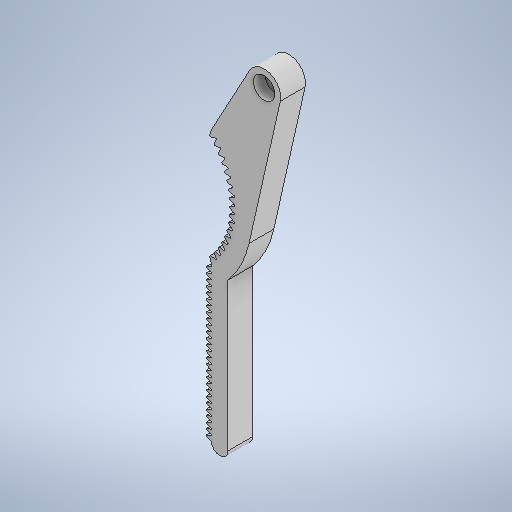
# Autodesk Inventor part: gripper_V2
Saved by Autodesk Inventor 2026.1 (Build 301233000, 233)
## iProperties
Created: 2025-11-11
Part Number: gripper_V2
Material: Generic
Document SubType Name: Modeling
Designer: kryst
Density: 1 g/cm^3
Appearance: Default
Author: kryst
Autodesk Inventor part; units mm, degrees
ref_plane "YZ Plane" through (0, 0, 0) normal (1, 0, 0) x (0, 1, 0)
ref_plane "XZ Plane" through (0, 0, 0) normal (0, 1, 0) x (-1, 0, 0)
ref_plane "XY Plane" through (0, 0, 0) normal (0, 0, 1) x (1, 0, 0)
sketch "Sketch1" plane through (0, 0, 0) normal (0, 0, 1) x (1, 0, 0)
  circle A0 centre (0, 0) radius 1.7
  circle A1 centre (0, 0) radius 3.25
  arc A2 (4.8776, -1.0993) -> (-4.3946, 2.3849) centre (0, 0) ccw
  line L0 (-16, -19) -> (-4.3946, 2.3849)
  arc A3 (-16, -54) -> (-16, -19) centre (-33.8536, -36.5) ccw
  line L1 (4.8776, -1.0993) -> (-4.5877, -43.096)
  line L2 (-10.3536, -36.25) -> (-10.3536, -36.75)
  line L3 (-10.3536, -36.75) -> (-8.8736, -37.5)
  line L4 (-10.3536, -36.25) -> (-8.8736, -35.5)
  line L5 (-10.475, -34.1008) -> (-9.0699, -33.2185)
  line L6 (-10.475, -34.1008) -> (-10.4293, -34.5987)
  line L7 (-10.4293, -34.5987) -> (-8.8869, -35.2101)
  line L8 (-10.4293, -38.4013) -> (-8.8869, -37.7899)
  line L9 (-10.4293, -38.4013) -> (-10.475, -38.8992)
  line L10 (-10.475, -38.8992) -> (-9.0699, -39.7815)
  line L11 (-10.7926, -31.9717) -> (-9.4741, -30.9645)
  line L12 (-10.7926, -31.9717) -> (-10.7015, -32.4633)
  line L13 (-10.7015, -32.4633) -> (-9.1096, -32.931)
  line L14 (-10.7015, -40.5367) -> (-9.1096, -40.069)
  line L15 (-10.7015, -40.5367) -> (-10.7926, -41.0283)
  line L16 (-10.7926, -41.0283) -> (-9.4741, -42.0355)
  line L17 (-11.3037, -29.8805) -> (-10.0829, -28.757)
  line L18 (-11.3037, -29.8805) -> (-11.168, -30.3618)
  line L19 (-11.168, -30.3618) -> (-9.54, -30.6819)
  line L20 (-11.168, -42.6382) -> (-9.54, -42.3181)
  line L21 (-11.168, -42.6382) -> (-11.3037, -43.1195)
  line L22 (-11.3037, -43.1195) -> (-10.0829, -44.243)
  line L23 (-12.004, -27.845) -> (-10.8911, -26.6144)
  line L24 (-12.004, -27.845) -> (-11.8248, -28.3117)
  line L25 (-11.8248, -28.3117) -> (-10.1744, -28.4816)
  line L26 (-11.8248, -44.6883) -> (-10.1744, -44.5184)
  line L27 (-11.8248, -44.6883) -> (-12.004, -45.155)
  line L28 (-12.004, -45.155) -> (-10.8911, -46.3856)
  line L29 (-12.8876, -25.882) -> (-11.892, -24.5548)
  line L30 (-12.8876, -25.882) -> (-12.6665, -26.3304)
  line L31 (-12.6665, -26.3304) -> (-11.0074, -26.3485)
  line L32 (-12.6665, -46.6696) -> (-11.0074, -46.6515)
  line L33 (-12.6665, -46.6696) -> (-12.8876, -47.118)
  line L34 (-12.8876, -47.118) -> (-11.892, -48.4452)
  line L35 (-13.9472, -24.0081) -> (-13.0771, -22.5954)
  line L36 (-13.9472, -24.0081) -> (-13.6859, -24.4344)
  line L37 (-13.6859, -24.4344) -> (-12.0321, -24.3006)
  line L38 (-13.6859, -48.5656) -> (-12.0321, -48.6994)
  line L39 (-13.6859, -48.5656) -> (-13.9472, -48.9919)
  line L40 (-13.9472, -48.9919) -> (-13.0771, -50.4047)
  line L41 (-15.1737, -22.2391) -> (-14.4366, -20.7526)
  line L42 (-15.1737, -22.2391) -> (-14.8745, -22.6397)
  line L43 (-14.8745, -22.6397) -> (-13.2399, -22.3551)
  line L44 (-14.8745, -50.3603) -> (-13.2399, -50.6449)
  line L45 (-14.8745, -50.3603) -> (-15.1737, -50.7609)
  line L46 (-15.1737, -50.7609) -> (-14.4366, -52.2474)
  line L47 (-16.557, -20.5896) -> (-15.9589, -19.042)
  line L48 (-16.557, -20.5896) -> (-16.2224, -20.9612)
  line L49 (-16.2224, -20.9612) -> (-14.6207, -20.5283)
  line L50 (-16.2224, -52.0388) -> (-14.6207, -52.4717)
  line L51 (-16.2224, -52.0388) -> (-16.557, -52.4104)
  line L52 (-16.557, -52.4104) -> (-15.9589, -53.958)
  line L53 (-15.9589, -53.958) -> (-15.9589, -100.657)
  line L54 (-15.9589, -53.958) -> (30.74, -53.958) construction
  arc A4 (-15.9589, -100.657) -> (-10.9589, -100.657) centre (-13.4589, -100.657) ccw
  line L55 (-17.4589, -99.732) -> (-17.4589, -100.082)
  line L56 (-17.4589, -100.082) -> (-15.9589, -100.657)
  line L57 (-17.4589, -99.732) -> (-15.9589, -99.157)
  line L58 (-17.4589, -98.032) -> (-15.9589, -97.457)
  line L59 (-17.4589, -98.032) -> (-17.4589, -98.382)
  line L60 (-17.4589, -98.382) -> (-15.9589, -98.957)
  line L61 (-17.4589, -96.332) -> (-15.9589, -95.757)
  line L62 (-17.4589, -96.332) -> (-17.4589, -96.682)
  line L63 (-17.4589, -96.682) -> (-15.9589, -97.257)
  line L64 (-17.4589, -94.632) -> (-15.9589, -94.057)
  line L65 (-17.4589, -94.632) -> (-17.4589, -94.982)
  line L66 (-17.4589, -94.982) -> (-15.9589, -95.557)
  line L67 (-17.4589, -92.932) -> (-15.9589, -92.357)
  line L68 (-17.4589, -92.932) -> (-17.4589, -93.282)
  line L69 (-17.4589, -93.282) -> (-15.9589, -93.857)
  line L70 (-17.4589, -91.232) -> (-15.9589, -90.657)
  line L71 (-17.4589, -91.232) -> (-17.4589, -91.582)
  line L72 (-17.4589, -91.582) -> (-15.9589, -92.157)
  line L73 (-17.4589, -89.532) -> (-15.9589, -88.957)
  line L74 (-17.4589, -89.532) -> (-17.4589, -89.882)
  line L75 (-17.4589, -89.882) -> (-15.9589, -90.457)
  line L76 (-17.4589, -87.832) -> (-15.9589, -87.257)
  line L77 (-17.4589, -87.832) -> (-17.4589, -88.182)
  line L78 (-17.4589, -88.182) -> (-15.9589, -88.757)
  line L79 (-17.4589, -86.132) -> (-15.9589, -85.557)
  line L80 (-17.4589, -86.132) -> (-17.4589, -86.482)
  line L81 (-17.4589, -86.482) -> (-15.9589, -87.057)
  line L82 (-17.4589, -84.432) -> (-15.9589, -83.857)
  line L83 (-17.4589, -84.432) -> (-17.4589, -84.782)
  line L84 (-17.4589, -84.782) -> (-15.9589, -85.357)
  line L85 (-17.4589, -82.732) -> (-15.9589, -82.157)
  line L86 (-17.4589, -82.732) -> (-17.4589, -83.082)
  line L87 (-17.4589, -83.082) -> (-15.9589, -83.657)
  line L88 (-17.4589, -81.032) -> (-15.9589, -80.457)
  line L89 (-17.4589, -81.032) -> (-17.4589, -81.382)
  line L90 (-17.4589, -81.382) -> (-15.9589, -81.957)
  line L91 (-17.4589, -79.332) -> (-15.9589, -78.757)
  line L92 (-17.4589, -79.332) -> (-17.4589, -79.682)
  line L93 (-17.4589, -79.682) -> (-15.9589, -80.257)
  line L94 (-17.4589, -77.632) -> (-15.9589, -77.057)
  line L95 (-17.4589, -77.632) -> (-17.4589, -77.982)
  line L96 (-17.4589, -77.982) -> (-15.9589, -78.557)
  line L97 (-17.4589, -75.932) -> (-15.9589, -75.357)
  line L98 (-17.4589, -75.932) -> (-17.4589, -76.282)
  line L99 (-17.4589, -76.282) -> (-15.9589, -76.857)
  line L100 (-17.4589, -74.232) -> (-15.9589, -73.657)
  line L101 (-17.4589, -74.232) -> (-17.4589, -74.582)
  line L102 (-17.4589, -74.582) -> (-15.9589, -75.157)
  line L103 (-17.4589, -72.532) -> (-15.9589, -71.957)
  line L104 (-17.4589, -72.532) -> (-17.4589, -72.882)
  line L105 (-17.4589, -72.882) -> (-15.9589, -73.457)
  line L106 (-17.4589, -70.832) -> (-15.9589, -70.257)
  line L107 (-17.4589, -70.832) -> (-17.4589, -71.182)
  line L108 (-17.4589, -71.182) -> (-15.9589, -71.757)
  line L109 (-17.4589, -69.132) -> (-15.9589, -68.557)
  line L110 (-17.4589, -69.132) -> (-17.4589, -69.482)
  line L111 (-17.4589, -69.482) -> (-15.9589, -70.057)
  line L112 (-17.4589, -67.432) -> (-15.9589, -66.857)
  line L113 (-17.4589, -67.432) -> (-17.4589, -67.782)
  line L114 (-17.4589, -67.782) -> (-15.9589, -68.357)
  line L115 (-17.4589, -65.732) -> (-15.9589, -65.157)
  line L116 (-17.4589, -65.732) -> (-17.4589, -66.082)
  line L117 (-17.4589, -66.082) -> (-15.9589, -66.657)
  line L118 (-10.9589, -100.657) -> (-10.9589, -55.8865)
  arc A5 (-10.9589, -55.8865) -> (-4.5877, -43.096) centre (-33.8536, -36.5) ccw
  line L119 (-17.4589, -64.032) -> (-15.9589, -63.457)
  line L120 (-17.4589, -64.032) -> (-17.4589, -64.382)
  line L121 (-17.4589, -64.382) -> (-15.9589, -64.957)
  line L122 (-17.4589, -62.332) -> (-15.9589, -61.757)
  line L123 (-17.4589, -62.332) -> (-17.4589, -62.682)
  line L124 (-17.4589, -62.682) -> (-15.9589, -63.257)
  line L125 (-17.4589, -60.632) -> (-15.9589, -60.057)
  line L126 (-17.4589, -60.632) -> (-17.4589, -60.982)
  line L127 (-17.4589, -60.982) -> (-15.9589, -61.557)
  line L128 (-17.4589, -58.932) -> (-15.9589, -58.357)
  line L129 (-17.4589, -58.932) -> (-17.4589, -59.282)
  line L130 (-17.4589, -59.282) -> (-15.9589, -59.857)
  line L131 (-17.4589, -57.232) -> (-15.9589, -56.657)
  line L132 (-17.4589, -57.232) -> (-17.4589, -57.582)
  line L133 (-17.4589, -57.582) -> (-15.9589, -58.157)
  line L134 (-17.4589, -55.532) -> (-15.9589, -54.957)
  line L135 (-17.4589, -55.532) -> (-17.4589, -55.882)
  line L136 (-17.4589, -55.882) -> (-15.9589, -56.457)
  point P0 (-8.8536, -36.5)
  point P1 (-10.3536, -36.5)
  point P2 (-8.9584, -34.2125)
  point P3 (-10.4522, -34.3497)
  point P4 (-8.9584, -38.7875)
  point P5 (-10.4522, -38.6503)
  point P6 (-9.2722, -31.9441)
  point P7 (-10.7471, -32.2175)
  point P8 (-9.2722, -41.0559)
  point P9 (-10.7471, -40.7825)
  point P10 (-9.7922, -29.714)
  point P11 (-11.2359, -30.1211)
  point P12 (-9.7922, -43.286)
  point P13 (-11.2359, -42.8789)
  point P14 (-10.5141, -27.5408)
  point P15 (-11.9144, -28.0784)
  point P16 (-10.5141, -45.4592)
  point P17 (-11.9144, -44.9216)
  point P18 (-11.4318, -25.4428)
  point P19 (-12.7771, -26.1062)
  point P20 (-11.4318, -47.5572)
  point P21 (-12.7771, -46.8938)
  point P22 (-12.5376, -23.4375)
  point P23 (-13.8165, -24.2213)
  point P24 (-12.5376, -49.5625)
  point P25 (-13.8165, -48.7787)
  point P26 (-13.8222, -21.5419)
  point P27 (-15.0241, -22.4394)
  point P28 (-13.8222, -51.4581)
  point P29 (-15.0241, -50.5606)
  point P30 (-15.275, -19.7717)
  point P31 (-16.3897, -20.7754)
  point P32 (-15.275, -53.2283)
  point P33 (-16.3897, -52.2246)
  point P34 (-17.4589, -99.907)
  point P35 (-17.4589, -98.207)
  point P36 (-17.4589, -96.507)
  point P37 (-17.4589, -94.807)
  point P38 (-17.4589, -93.107)
  point P39 (-17.4589, -91.407)
  point P40 (-17.4589, -89.707)
  point P41 (-17.4589, -88.007)
  point P42 (-17.4589, -86.307)
  point P43 (-17.4589, -84.607)
  point P44 (-17.4589, -82.907)
  point P45 (-17.4589, -81.207)
  point P46 (-17.4589, -79.507)
  point P47 (-17.4589, -77.807)
  point P48 (-17.4589, -76.107)
  point P49 (-17.4589, -74.407)
  point P50 (-17.4589, -72.707)
  point P51 (-17.4589, -71.007)
  point P52 (-17.4589, -69.307)
  point P53 (-17.4589, -67.607)
  point P54 (-17.4589, -65.907)
  point P55 (-15.9589, -65.157)
  point P56 (-15.9589, -66.657)
  point P57 (-15.9589, -66.857)
  point P58 (-15.9589, -68.357)
  point P59 (-15.9589, -68.557)
  point P60 (-15.9589, -70.057)
  point P61 (-15.9589, -70.257)
  point P62 (-15.9589, -71.757)
  point P63 (-15.9589, -71.957)
  point P64 (-15.9589, -73.457)
  point P65 (-15.9589, -73.657)
  point P66 (-15.9589, -75.157)
  point P67 (-15.9589, -75.357)
  point P68 (-15.9589, -76.857)
  point P69 (-15.9589, -77.057)
  point P70 (-15.9589, -78.557)
  point P71 (-15.9589, -78.757)
  point P72 (-15.9589, -80.257)
  point P73 (-15.9589, -80.457)
  point P74 (-15.9589, -81.957)
  point P75 (-15.9589, -82.157)
  point P76 (-15.9589, -83.657)
  point P77 (-15.9589, -83.857)
  point P78 (-15.9589, -85.357)
  point P79 (-15.9589, -85.557)
  point P80 (-15.9589, -87.057)
  point P81 (-15.9589, -87.257)
  point P82 (-15.9589, -88.757)
  point P83 (-15.9589, -88.957)
  point P84 (-15.9589, -90.457)
  point P85 (-15.9589, -90.657)
  point P86 (-15.9589, -92.157)
  point P87 (-15.9589, -92.357)
  point P88 (-15.9589, -93.857)
  point P89 (-15.9589, -94.057)
  point P90 (-15.9589, -95.557)
  point P91 (-15.9589, -95.757)
  point P92 (-15.9589, -97.257)
  point P93 (-15.9589, -97.457)
  point P94 (-15.9589, -98.957)
  point P95 (-17.4589, -64.207)
  point P96 (-17.4589, -62.507)
  point P97 (-17.4589, -60.807)
  point P98 (-17.4589, -59.107)
  point P99 (-17.4589, -57.407)
  point P100 (-17.4589, -55.707)
  point P101 (-15.9589, -64.957)
  point P102 (-15.9589, -63.457)
  point P103 (-15.9589, -63.257)
  point P104 (-15.9589, -61.757)
  point P105 (-15.9589, -61.557)
  point P106 (-15.9589, -60.057)
  point P107 (-15.9589, -59.857)
  point P108 (-15.9589, -58.357)
  point P109 (-15.9589, -58.157)
  point P110 (-15.9589, -56.657)
  point P111 (-15.9589, -56.457)
  point P112 (-15.9589, -54.957)
  dimension "d10" = 25
  dimension "d0" = 3.4
  dimension "d1" = 6.5
  dimension "d2" = 10
  dimension "d9" = 35
  dimension "d14" = 0.5
  dimension "d15" = 2
  dimension "d16" = 1.5
  dimension "d17" = 1.48
  dimension "d24" = 84
  dimension "d36" = 21.3849
  dimension "d37" = 19
  dimension "d38" = 41.9967
  dimension "d39" = 1.0993
  dimension "d44" = 0.35
  dimension "d45" = 1.5
  dimension "d47" = 1.5
  dimension "d49" = 0.575
  dimension "d52" = 1.7
  dimension "d64" = 2.5
  dimension "d65" = 44.7705
  constraints: 272 end point, 131 vertical alignment, 52 parallel, 26 collinear, 6 point on circle, 5 centre point, 4 coincident, 4 tangent, 3 vertical, 2 equal length, 2 horizontal, 2 midpoint, 1 horizontal alignment, 156 other
  measures "d0" diameter of A0
  measures "d1" diameter of A1
  measures "d2" diameter of A2
  measures "d9" distance of L0.start point (-16, -54)
  measures "d14" distance of L2.start L2.end
  measures "d15" distance of L3.end L4.end
  measures "d16" distance of point (-8.854, -36.5) point (-10.354, -36.5)
  measures "d17" horizontal distance of L2.start L4.end
  measures "d36" vertical distance of L0.end L0.start
  measures "d37" vertical distance of L0.start point (0, 0)
  measures "d38" vertical distance of L1.start L1.end
  measures "d39" vertical distance of L1.start point (0, 0)
  measures "d44" distance of L57.start L55.end
  measures "d45" distance of L56.end L57.end
  measures "d47" horizontal distance of L57.start L57.end
  measures "d49" vertical distance of L57.start L57.end
  measures "d52" distance of L57.end L58.end
  measures "d64" radius of A4
  measures "d65" distance of L118.start L118.end
extrude "Extrusion1" add sketch "Sketch1" along normal blind 7.5 contours L1 A5 L118 A4 L53 A3 L0 A2 | A3 L49 L48 L47 | L56 L55 L57 L53 | A3 L43 L42 L41 | L60 L59 L58 L53 | A3 L37 L36 L35 | L63 L62 L61 L53 | A3 L31 L30 L29 | L66 L65 L64 L53 | A3 L25 L24 L23 | L69 L68 L67 L53 | A3 L19 L18 L17 | L72 L71 L70 L53 | A3 L13 L12 L11 | L75 L74 L73 L53 | A3 L7 L6 L5 | L78 L77 L76 L53 | A3 L3 L2 L4 | L81 L80 L79 L53 | A3 L10 L9 L8 | L84 L83 L82 L53 | A3 L16 L15 L14 | L87 L86 L85 L53 | A3 L22 L21 L20 | L90 L89 L88 L53 | A3 L28 L27 L26 | L93 L92 L91 L53 | A3 L34 L33 L32 | L96 L95 L94 L53 | A3 L40 L39 L38 | L99 L98 L97 L53 | A3 L46 L45 L44 | L102 L101 L100 L53 | A3 L52 L51 L50 | L105 L104 L103 L53 | L53 L136 L135 L134 | L108 L107 L106 L53 | L53 L133 L132 L131 | L111 L110 L109 L53 | L53 L130 L129 L128 | L114 L113 L112 L53 | L53 L127 L126 L125 | L117 L116 L115 L53 | L53 L124 L123 L122 | L121 L120 L119 L53
extrude "Extrusion2" add sketch "Sketch1" along normal blind 4 contours A1
body "Solid1"
